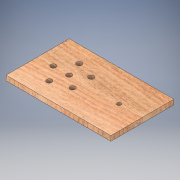
# Autodesk Inventor part: Stage3Wall
Saved by Autodesk Inventor 2017 (Build 210142000, 142)
## iProperties
Created: 2017-02-01
Part Number: Stage3Wall
Material: Wood (Birch)
Document SubType Name: Modeling
Designer: Naga
Density: 0.55 g/cm^3
Appearance: Birch - Natural Polished
Author: Naga
Autodesk Inventor part; units mm, degrees
ref_plane "YZ Plane" through (0, 0, 0) normal (1, 0, 0) x (0, 1, 0)
ref_plane "XZ Plane" through (0, 0, 0) normal (0, 1, 0) x (-1, 0, 0)
ref_plane "XY Plane" through (0, 0, 0) normal (0, 0, 1) x (1, 0, 0)
sketch "Sketch1" plane through (0, 0, 0) normal (0, 1, 0) x (-1, 0, 0)
  line L0 (0, 0) -> (253.2063, 0)
  line L1 (253.2063, 0) -> (253.2063, -152.4)
  line L2 (253.2063, -152.4) -> (0, -152.4)
  line L3 (0, -152.4) -> (0, 0)
  line L4 (0, -76.2) -> (56.3563, -76.2)
  circle A0 centre (56.3563, -76.2) radius 4.7625
  dimension "d0" = 152.4
  dimension "d1" = 253.2063
  dimension "d2" = 56.3563
  dimension "d3" = 9.525
  constraints: 10 end point, 2 horizontal, 2 parallel, 1 centre point, 1 coincident, 1 midpoint, 1 perpendicular
  measures "d0" distance of L2.end L0.start
  measures "d1" distance of L0.start L0.end
  measures "d2" distance of L4.start L4.end
  measures "d3" diameter of A0
extrude "Extrusion1" add sketch "Sketch1" along normal blind 11.9062
sketch "Sketch2" plane through (0, 11.9062, 0) normal (0, 1, 0) x (1, 0, 0)
  line L0 (0, 0) -> (0, 152.4) projected
  line L1 (0, 76.2) -> (-177.0063, 76.2)
  circle A0 centre (-177.0063, 76.2) radius 6.35
  line L2 (-177.0063, 76.2) -> (-215.1063, 76.2)
  circle A1 centre (-215.1063, 76.2) radius 6.35
  circle A2 centre (-188.7798, 39.9647) radius 6.35
  circle A3 centre (-146.1827, 53.8054) radius 6.35
  circle A4 centre (-146.1827, 98.5946) radius 6.35
  circle A5 centre (-188.7798, 112.4353) radius 6.35
  dimension "d6" = 12.7
  dimension "d7" = 38.1
  dimension "d8" = 12.7
  dimension "d11" = 360
  dimension "d13" = 177.0062
  constraints: 6 centre point, 4 end point, 2 coincident, 2 horizontal, 1 midpoint, 11 other
  measures "d6" diameter of A0
  measures "d7" distance of L2.start L2.end
  measures "d8" diameter of A1
  measures "d13" distance of L1.start L1.end
extrude "Extrusion2" cut sketch "Sketch2" against normal blind 11.9062
body "Solid1"
